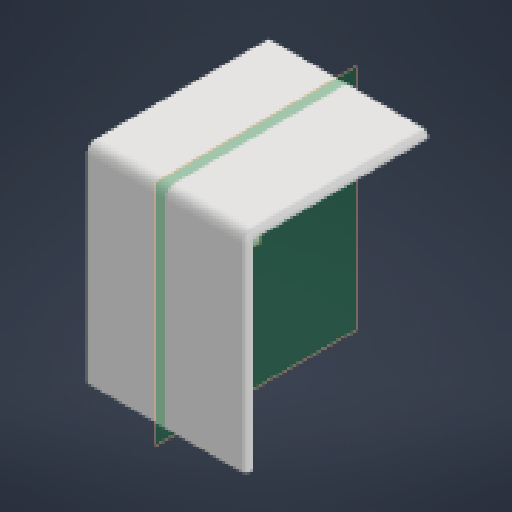
# Autodesk Inventor part: tail_box_cup
Saved by Autodesk Inventor 2024 (Build 280153000, 153)
## iProperties
Created: 2023-05-16
Part Number: tail_box_cup
Material: Типовые
Document SubType Name: Modeling
Designer: user
Density: 1 g/cm^3
Appearance: По умолчанию
Author: user
Autodesk Inventor part; units mm, degrees
ref_plane "YZ Plane" through (0, 0, 0) normal (1, 0, 0) x (0, 1, 0)
ref_plane "XZ Plane" through (0, 0, 0) normal (0, 1, 0) x (-1, 0, 0)
ref_plane "XY Plane" through (0, 0, 0) normal (0, 0, 1) x (1, 0, 0)
sketch "Эскиз1" plane through (0, 0, 0) normal (0, 0, 1) x (1, 0, 0)
  line L0 (28.5, 35) -> (-28.5, 35)
  arc A0 (32.5, 31) -> (28.5, 35) centre (28.5, 31) ccw
  arc A1 (-28.5, 35) -> (-32.5, 31) centre (-28.5, 31) ccw
  line L1 (-32.5, 31) -> (-32.5, -35)
  line L2 (32.5, -35) -> (32.5, 31)
  line L3 (26.5, -35) -> (32.5, -35)
  line L4 (-32.5, -35) -> (-26.5, -35)
  line L5 (26.5, -35) -> (-26.5, -35)
  point P0 (0, 0)
extrude "Выдавливание1" add sketch "Эскиз1" along normal blind 3
ref_plane "РабПлоскость1" through (26.5, -31, -4) normal (-1, 0, 0) x (0, -1, 0)
sketch "Эскиз3" plane through (26.5, -31, -4) normal (-1, 0, 0) x (0, -1, 0)
  line L0 (-4, 4) -> (-4, -4) projected
  line L1 (-4, -4) -> (4, -4) projected
  line L2 (4, -4) -> (4, 4) projected
  line L3 (4, 4) -> (-4, 4) projected
  circle A0 centre (0, 0) radius 1.95 projected
  point P0 (-31, 4)
extrude "Выдавливание3" add sketch "Эскиз3" along normal blind 5
sketch "Эскиз4" plane through (-32.5, -35, 3) normal (0, -1, 0) x (1, 0, 0)
  line L0 (0, -79.5) -> (0, -3) projected
  line L1 (0, -3) -> (0, 0) projected
  line L2 (0, 0) -> (65, 0) projected
  line L3 (65, -3) -> (65, 0) projected
  line L4 (65, -79.5) -> (65, -3) projected
  arc A0 (61, -83.5) -> (65, -79.5) centre (61, -79.5) ccw projected
  line L5 (4, -83.5) -> (61, -83.5) projected
  arc A1 (0, -79.5) -> (4, -83.5) centre (4, -79.5) ccw projected
  point P0 (32.5, -3)
extrude "Выдавливание4" add sketch "Эскиз4" along normal blind 3
ref_plane "РабПлоскость3" through (0, 31, 0) normal (-1, 0, 0) x (0, 0, 1)
mirror "Зеркальное отражение2" about plane through (0, 31, 0) normal (-1, 0, 0) of "Выдавливание3"
fillet "Сопряжение3" radius 4 1 edges at (0, -38, 3)
